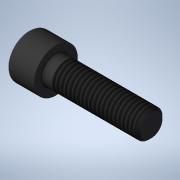
# Autodesk Inventor part: Slotted head cap screw ISO 4762 - M10x35
Saved by Autodesk Inventor 2021 (Build 250183000, 183)
## iProperties
Created: 2025-07-30
Part Number: Slotted head cap screw ISO 4762 - M10x35
Material: Generic
Catalog Web Link: www.cadenas.de
Description: ISO 4762-Hexagon socket head cap screw
Vendor: SCHUNK
Document SubType Name: Modeling
Designer: psAdmin
Manufacturer: SCHUNK
Mass: 4.41015 g
Surface Area: 21.202 cm^2
Volume: 4.41015 cm^3
Density: 1 g/cm^3
Appearance: PSOLRGB-175-175-175
Category: PARTsolutions
Company: SCHUNK
Title: Slotted head cap screw ISO 4762 - M10x35
Author: Cadenas PARTsolutions
Comments: Hexagon socket head cap screw
PSOL_IDENT_0: {$CADENAS_DATA/23d-libs/schunk/normteile/din_en_iso_4762.prj},239 {M=Nenngewinde},{VTYP=3D},{NB=Slot
PSOL_IDENT_1: ted head cap screw ISO 4762 - M10x35},{LINA=Slotted head cap screw ISO 4762 - M10x35},{NN=ISO 4762},
PSOL_IDENT_2: {DATE=16.11.2022 07:48:45},{GEOMDATE=14.11.2022 10:51:17},{VERSION=},{LINEID=880},{WBVAR=},{WBNUMERI
PSOL_IDENT_3: C=}  {NB=Zylinderschraube ISO 4762 - M10x35},{LINA=Zylinderschraube ISO 4762 - M10x35},{KT=DUMMY},{I
PSOL_IDENT_4: DNR=},{D=10.000},{L=35.000},{D3=8.160},{P=1.500},{B=35.000},{S=8.000},{DK=16.000},{DA=11.200},{DS=10
PSOL_IDENT_5: .000},{E=9.150},{K=10.000},{R=0.400},{T=5.000},{V=1.000},{DW=15.330},{W=4.000},{LF=1.020},{LG=4.500}
PSOL_IDENT_6: ,{FORM=1.000},{ASG=0.000},{SDMODELL1=0.000},{NENN=M10x35},{TYP=90.000}
NB: Slotted head cap screw ISO 4762 - M10x35
NN: ISO 4762
NT: Hexagon socket head cap screw
NBSYN: Slotted head cap screw ISO 4762 - $NENN.
LINA: Slotted head cap screw ISO 4762 - M10x35
CATALOG: SCHUNK
ROWDESC: M10x35
D: 10
L: 35
D3: 8.16
P: 1.5
B: 35
S: 8
DK: 16
DA: 11.2
DS: 10
E: 9.15
K: 10
R: 0.4
T: 5
V: 1
DW: 15.33
W: 4
LF: 1.02
LG: 4.5
FORM: 1
ASG: 0
SDMODELL1: 0
TYP: 90
SUPPLIER: SCHUNK
ARTICLENO: Slotted head cap screw ISO 4762 - M10x35
BOMINFO: Slotted head cap screw ISO 4762 - M10x35
CREATOR: CADENAS GmbH
Autodesk Inventor part; units mm, degrees
sketch "Skizze_2" plane through (0, 0, 0) normal (0, 0, 1) x (1, 0, 0)
  line L0 (38, 0) -> (-10, 0)
  line L1 (-10, 0) -> (-10, 7)
  arc A0 (-9, 8) -> (-10, 7) centre (-9, 7) ccw
  line L2 (-9, 8) -> (0, 8)
  line L3 (0, 8) -> (0, 5.6)
  arc A1 (0, 5.6) -> (0.2772, 5.2193) centre (0.4, 5.6) ccw
  line L4 (0.2772, 5.2193) -> (0.8972, 5.0193)
  arc A2 (0.8972, 5.0193) -> (1.02, 5) centre (1.02, 5.4) ccw
  line L5 (1.02, 5) -> (34.08, 5)
  line L6 (34.08, 5) -> (35, 4.08)
  line L7 (35, 4.08) -> (35, 0)
  line L8 (35, 0) -> (-10, 0)
  constraints: 18 end point, 6 point on circle, 3 centre point
revolve "Revolution1" add sketch "Skizze_2" angle 360 about axis through (38, 0, 0) along (1, 0, 0)
thread "Thread1" size "M10x1.5" class "6g" standard "ISO Metric profile" length 30.5
sketch "Skizze_1" plane through (-4.001, 0, 0) normal (1, 0, 0) x (0, 0, -1)
  line L0 (-3.995, -2.3065) -> (0, -4.613)
  line L1 (0, -4.613) -> (3.995, -2.3065)
  line L2 (3.995, -2.3065) -> (3.995, 2.3065)
  line L3 (3.995, 2.3065) -> (0, 4.613)
  line L4 (0, 4.613) -> (-3.995, 2.3065)
  line L5 (-3.995, 2.3065) -> (-3.995, -2.3065)
  constraints: 12 end point
extrude "Extrusion1" cut sketch "Skizze_1" against normal blind 10.01
ref_plane "IP1_XY" through (0, 0, 0) normal (1, 0, 0) x (0, 0, -1)
ref_plane "IP1_YZ" through (0, 0, 0) normal (0, 0, -1) x (0, 1, 0)
ref_plane "IP1_ZX" through (0, 0, 0) normal (0, 1, 0) x (1, 0, 0)
ref_plane "IP2_XY" through (-10, 0, 0) normal (1, 0, 0) x (0, 0, -1)
ref_plane "IP2_YZ" through (-10, 0, 0) normal (0, 0, -1) x (0, 1, 0)
ref_plane "IP2_ZX" through (-10, 0, 0) normal (0, 1, 0) x (1, 0, 0)
ref_plane "IP3_XY" through (35, 0, 0) normal (1, 0, 0) x (0, 0, -1)
ref_plane "IP3_YZ" through (35, 0, 0) normal (0, 0, -1) x (0, 1, 0)
ref_plane "IP3_ZX" through (35, 0, 0) normal (0, 1, 0) x (1, 0, 0)
body "Solid1"
